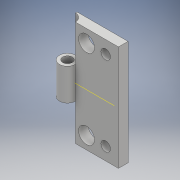
# Autodesk Inventor part: k2_hinge1_top
Saved by Autodesk Inventor 2017 (Build 210142000, 142)
## iProperties
Created: 2017-02-14
Part Number: k2_hinge1_top
Material: Generic
Document SubType Name: Modeling
Designer: herman
Density: 1 g/cm^3
Appearance: Default
Author: herman
Autodesk Inventor part; units mm, degrees
ref_plane "YZ Plane" through (0, 0, 0) normal (1, 0, 0) x (0, 1, 0)
ref_plane "XZ Plane" through (0, 0, 0) normal (0, 1, 0) x (-1, 0, 0)
ref_plane "XY Plane" through (0, 0, 0) normal (0, 0, 1) x (1, 0, 0)
sketch "Sketch1" plane through (0, 0, 0) normal (0, 1, 0) x (-1, 0, 0)
  line L0 (9.6232, 12.9345) -> (-6.3768, 12.9345)
  line L1 (-6.3768, 12.9345) -> (-6.3768, -20.0655)
  line L2 (-6.3768, -20.0655) -> (9.6232, -20.0655)
  line L3 (9.6232, -20.0655) -> (9.6232, 12.9345)
  dimension "d3" = 16
  dimension "d4" = 33
  constraints: 8 end point, 2 parallel, 1 horizontal, 1 perpendicular
  measures "d3" distance of L0.start L0.end
  measures "d4" distance of L2.end L0.start
extrude "Extrusion1" add sketch "Sketch1" along normal blind 3
sketch "Sketch2" plane through (0, 3, 0) normal (0, 1, 0) x (1, 0, 0)
  circle A0 centre (2.3768, -8.9345) radius 1.5
  circle A1 centre (2.3768, 16.0655) radius 1.5
  line L0 (6.3768, -12.9345) -> (6.3768, 20.0655) projected
  line L1 (-9.6232, -12.9345) -> (6.3768, -12.9345) projected
  line L2 (6.3768, 20.0655) -> (-9.6232, 20.0655) projected
  point P0 (0, 0)
  dimension "d7" = 3
  dimension "d8" = 3
  dimension "d9" = 4
  dimension "d10" = 4
  dimension "d11" = 4
  dimension "d12" = 4
  constraints: 2 centre point
  measures "d7" diameter of A0
  measures "d8" diameter of A1
  measures "d9" distance from line of L0 A0.centre
  measures "d10" distance from line of L1 A0.centre
  measures "d11" distance from line of L0 A1.centre
  measures "d12" distance from line of L2 A1.centre
extrude "Extrusion2" cut sketch "Sketch2" against normal through all
ref_plane "Work Plane1" through (-9.6232, 0, -3.5655) normal (0, 0, 1) x (1, 0, 0)
sketch "Sketch4" plane through (-9.6232, 0, -3.5655) normal (0, 0, 1) x (1, 0, 0)
  line L0 (0, 0) -> (0, 3) projected
  circle A0 centre (0, 0) radius 2.5
  point P0 (9.6232, 0)
  dimension "d17" = 5
  constraints: 1 centre point
  measures "d17" diameter of A0
extrude "Extrusion3" add sketch "Sketch4" along normal mid plane 10
sketch "Sketch5" plane through (-9.6232, 0, 12.9345) normal (0, 0, 1) x (1, 0, 0)
  line L0 (0, 2.5) -> (0, 0) projected
  circle A0 centre (0, 0) radius 2.5
  point P0 (9.6232, 0)
  dimension "d21" = 5
  constraints: 1 centre point
  measures "d21" diameter of A0
extrude "Extrusion4" cut sketch "Sketch5" against normal blind 11.5
mirror "Mirror1" about plane through (-9.6232, 0, -3.5655) normal (0, 0, 1) of "Extrusion4"
sketch "Sketch6" plane through (-9.6232, 0, 1.4345) normal (0, 0, 1) x (1, 0, 0)
  circle A0 centre (0, 0) radius 1.5
  point P0 (9.6232, 0)
  dimension "d24" = 3
  constraints: 1 centre point
  measures "d24" diameter of A0
extrude "Extrusion5" cut sketch "Sketch6" against normal up to next
sketch "Sketch7" plane through (0, 0, 0) normal (0, -1, 0) x (1, 0, 0)
  circle A0 centre (-3.6232, -16.0655) radius 2.5
  circle A1 centre (-3.6232, 8.9345) radius 2.5
  line L0 (6.3768, -20.0655) -> (-7.1232, -20.0655) projected
  line L1 (-7.1232, 12.9345) -> (6.3768, 12.9345) projected
  line L2 (-7.1232, 12.9345) -> (-7.1232, 1.4345) projected
  point P0 (0, 0)
  dimension "d27" = 5
  dimension "d28" = 5
  dimension "d29" = 4
  dimension "d30" = 4
  dimension "d31" = 3.5
  dimension "d32" = 3.5
  constraints: 2 centre point
  measures "d27" diameter of A0
  measures "d28" diameter of A1
  measures "d29" distance from line of L0 A0.centre
  measures "d30" distance from line of L1 A1.centre
  measures "d31" horizontal distance of L1.start A1.centre
  measures "d32" horizontal distance of L0.end A0.centre
extrude "Extrusion6" cut sketch "Sketch7" against normal through all
equation "\"d11\" = d9"
equation "\"d12\" = d10"
equation "\"d30\" = d29"
equation "\"d32\" = d31"
body "Solid1"
